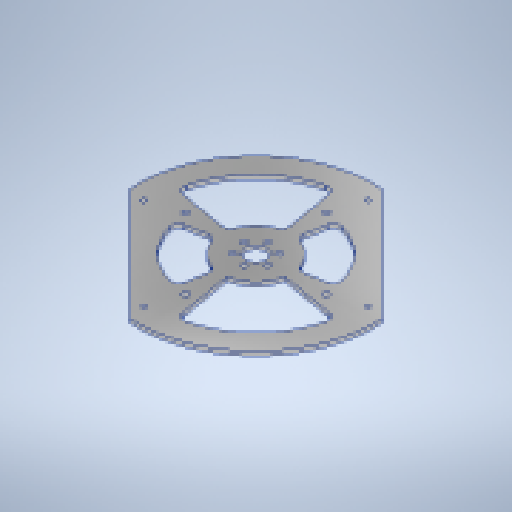
# Autodesk Inventor part: baseplate_R2toR6
Saved by Autodesk Inventor 2024.3 (Build 283343010, 343A)
## iProperties
Created: 2025-05-25
Part Number: baseplate_R2toR6
Material: アルミニウム 6061
Document SubType Name: Modeling
Designer: kshau
Density: 2.7 g/cm^3
Appearance: アルミニウム - フラット
Mass: 150.999 g
Surface Area: 394.685 cm^2
Volume: 55.9256 cm^3
Author: kshau
Autodesk Inventor part; units mm, degrees
ref_plane "YZ Plane" through (0, 0, 0) normal (1, 0, 0) x (0, 1, 0)
ref_plane "XZ Plane" through (0, 0, 0) normal (0, 1, 0) x (-1, 0, 0)
ref_plane "XY Plane" through (0, 0, 0) normal (0, 0, 1) x (1, 0, 0)
sketch "スケッチ1" plane through (0, 0, 0) normal (0, 1, 0) x (-1, 0, 0)
  circle A0 centre (0, 0) radius 86.2565
  circle A1 centre (0, 0) radius 7.5
  dimension "d0" = 172.513
  dimension "d1" = 15
  constraints: 2 centre point, 2 coincident
  measures "d0" diameter of A0
  measures "d1" diameter of A1
extrude "押し出し1" add sketch "スケッチ1" along normal blind 3
sketch "スケッチ2" plane through (0, 3, 0) normal (0, 1, 0) x (1, 0, 0)
  circle A0 centre (0, 0) radius 50.75
  point P0 (0, 50.75)
  point P1 (-50.75, 0)
  point P2 (0, -50.75)
  point P3 (50.75, 0)
  dimension "d4" = 101.5
  dimension "d7" = 360
  constraints: 1 coincident, 1 vertical alignment, 7 other
hole "穴1" at (0, 3, -50.75) at (-50.75, 3, 0) at (0, 3, 50.75) at (50.75, 3, 0) direction (0, -1, 0) diameter 4.3 end through all
sketch "スケッチ3" plane through (0, 3, 0) normal (0, 1, 0) x (1, 0, 0)
  line L0 (0, 0) -> (86.2565, 0)
  circle A0 centre (0, 0) radius 86.2565 projected
  circle A1 centre (0, 0) radius 7.5 projected
  line L1 (0, 0) -> (60.9926, -60.9926)
  line L2 (-8.1772, -85.868) -> (-85.868, -8.1772)
  line L3 (85.868, 8.1772) -> (8.1772, 85.868)
  point P0 (8.1772, 85.868)
  point P1 (83.085, 0)
  point P2 (85.868, 8.1772)
  dimension "d16" = 45
  dimension "d64" = 66.5
  constraints: 8 end point, 4 point on circle, 2 symmetric about line, 1 horizontal, 1 parallel
  measures "d16" angle of L0 L1
  measures "d64" distance between parallel lines of L2 L1
extrude "押し出し2" cut sketch "スケッチ3" against normal blind 3 contours L3 A0 | A0 L2
sketch "スケッチ4" plane through (0, 3, 0) normal (0, 1, 0) x (1, 0, 0)
  circle A0 centre (0, 0) radius 7.5 projected
  circle A1 centre (0, 0) radius 12
  line L0 (0, 0) -> (-8.4853, -8.4853)
  line L1 (0, 0) -> (-12, 0)
  point P0 (3.1058, -11.5911)
  point P1 (11.5911, -3.1058)
  point P2 (8.4853, 8.4853)
  point P3 (-3.1058, 11.5911)
  point P4 (-11.5911, 3.1058)
  dimension "d20" = 24
  dimension "d21" = 45
  dimension "d24" = 360
  constraints: 4 end point, 2 coincident, 2 point on circle, 1 centre point, 1 horizontal, 7 other
  measures "d20" diameter of A1
  measures "d21" angle of L1 L0
hole "穴2" at (-8.4853, 3, 8.4853) at (3.1058, 3, 11.5911) at (11.5911, 3, 3.1058) at (8.4853, 3, -8.4853) at (-3.1058, 3, -11.5911) at (-11.5911, 3, -3.1058) direction (0, -1, 0) diameter 4.3 end through all
sketch "スケッチ5" plane through (0, 3, 0) normal (0, 1, 0) x (1, 0, 0)
  arc A0 (-8.1772, -85.868) -> (85.868, 8.1772) centre (0, 0) ccw projected
  line L0 (5.2626, -86.0958) -> (-86.0958, 5.2626)
  arc A1 (8.1772, 85.868) -> (-85.868, -8.1772) centre (0, 0) ccw projected
  line L1 (-85.868, -8.1772) -> (-8.1772, -85.868) projected
  line L2 (-5.2626, 86.0958) -> (86.0958, -5.2626)
  line L3 (85.868, 8.1772) -> (8.1772, 85.868) projected
  line L4 (-85.868, -8.1772) -> (8.1772, 85.868)
  line L5 (-8.1772, -85.868) -> (85.868, 8.1772)
  line L6 (-73.6506, -7.1826) -> (7.1826, 73.6506)
  line L7 (80.2566, 13.7886) -> (-7.1826, -73.6506)
  line L8 (0, 0) -> (40.4166, 40.4166)
  circle A2 centre (0, 0) radius 74
  point P0 (-73.6506, -7.1826)
  point P1 (7.1826, 73.6506)
  point P2 (73.6506, 7.1826)
  dimension "d61" = 148
  dimension "d62" = 47
  dimension "d63" = 47
  constraints: 14 end point, 6 point on circle, 6 point on line, 4 coincident, 4 perpendicular, 2 parallel, 1 centre point, 1 midpoint
  measures "d61" diameter of A2
  measures "d62" distance between parallel lines of L8 L6
  measures "d63" distance between parallel lines of L8 L7
hole "穴3" at (-73.6506, 3, 7.1826) at (7.1826, 3, -73.6506) at (73.6506, 3, -7.1826) at (-7.1826, 3, 73.6506) direction (0, -1, 0) diameter 3.2 end through all
sketch "スケッチ6" plane through (0, 3, 0) normal (0, 1, 0) x (1, 0, 0)
  circle A0 centre (0, 0) radius 7.5 projected
  circle A1 centre (0, 0) radius 70
  circle A2 centre (0, 0) radius 50
  circle A3 centre (7.1826, 73.6506) radius 1.6 projected
  line L0 (0, 0) -> (7.1826, 73.6506)
  circle A4 centre (-73.6506, -7.1826) radius 1.6 projected
  line L1 (0, 0) -> (-73.6506, -7.1826)
  line L2 (0, 0) -> (-11.469, 69.0541)
  line L3 (0, 0) -> (-69.0541, 11.469)
  circle A5 centre (0, 0) radius 25
  circle A6 centre (0, 50.75) radius 2.15 projected
  line L4 (0, 0) -> (0, 50.75)
  line L5 (0, 0) -> (8.6824, 49.2404)
  line L6 (0, 0) -> (49.2404, 8.6824)
  circle A7 centre (50.75, 0) radius 2.15 projected
  line L7 (0, 0) -> (50.75, 0)
  line L8 (0, 0) -> (-49.2404, -8.6824)
  line L9 (0, 0) -> (-8.6824, -49.2404)
  line L10 (0, 0) -> (11.469, -69.0541)
  line L11 (0, 0) -> (69.0541, -11.469)
  circle A8 centre (0, 0) radius 40
  point P0 (-4.3412, -24.6202)
  point P1 (-24.6202, -4.3412)
  point P2 (49.3243, -8.1921)
  point P3 (24.6622, -4.0961)
  point P4 (4.0961, -24.6622)
  point P5 (8.1921, -49.3243)
  point P6 (24.6202, 4.3412)
  point P7 (4.3412, 24.6202)
  point P8 (-24.6622, 4.0961)
  point P9 (-4.0961, 24.6622)
  point P10 (-8.1921, 49.3243)
  point P11 (-49.3243, 8.1921)
  point P12 (69.0541, -11.469)
  point P13 (11.469, -69.0541)
  point P14 (39.4595, -6.5537)
  point P15 (6.5537, -39.4595)
  point P16 (-39.4595, 6.5537)
  point P17 (-6.5537, 39.4595)
  dimension "d44" = 140
  dimension "d45" = 100
  dimension "d46" = 15
  dimension "d47" = 15
  dimension "d48" = 50
  dimension "d49" = 10
  dimension "d50" = 10
  dimension "d53" = 360
  dimension "d57" = 80
  constraints: 24 end point, 5 coincident, 4 centre point, 4 point on circle, 1 horizontal, 1 vertical, 21 other
  measures "d44" diameter of A1
  measures "d45" diameter of A2
  measures "d46" angle of L0 L2
  measures "d47" angle of L1 L3
  measures "d48" diameter of A5
  measures "d49" angle of L4 L5
  measures "d50" angle of L7 L6
  measures "d57" diameter of A8
extrude "押し出し3" cut sketch "スケッチ6" against normal blind 10 contours A5 L5 A8 L6 | L11 A8 L10 A5 | A8 L5 A2 L6 | L11 A2 L10 A8 | A5 L3 A8 L2 | A5 L9 A8 L8 | L11 A1 L10 A2 | A8 L3 A2 L2 | A8 L9 A2 L8 | A2 L3 A1 L2
fillet "フィレット1" radius 5 14 edges at (-11.469, 1.5, -69.0541) (-69.0541, 1.5, -11.469) (-49.2404, 1.5, 8.6824) (-24.6202, 1.5, 4.3412) (-8.6824, 1.5, 49.2404) (-4.3412, 1.5, 24.6202) (11.469, 1.5, 69.0541) (69.0541, 1.5, 11.469) (24.6202, 1.5, -4.3412) (49.2404, 1.5, -8.6824) (8.6824, 1.5, -49.2404) (4.3412, 1.5, -24.6202) (-4.0961, 1.5, -24.6622) (-24.6622, 1.5, -4.0961)
equation "\"d64\" = Almiwidth4"
equation "\"d62\" = Almiwidth1"
equation "\"d63\" = Almiwidth1"
equation "\"Almiwidth4\" = 66.5"
equation "\"Almiwidth1\" = 47"
